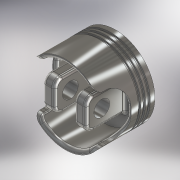
# Autodesk Inventor part: Piston head
Saved by Autodesk Inventor 2019 (Build 230136000, 136)
## iProperties
Created: 2020-05-28
Part Number: Piston head
Material: Generic
Document SubType Name: Modeling
Designer: Manoj
Density: 1 g/cm^3
Appearance: Chrome - Polished
Mass: 435.392 g
Surface Area: 893.496 cm^2
Volume: 435.392 cm^3
Author: Manoj
Autodesk Inventor part; units mm, degrees
ref_plane "YZ Plane" through (0, 0, 0) normal (1, 0, 0) x (0, 1, 0)
ref_plane "XZ Plane" through (0, 0, 0) normal (0, 1, 0) x (-1, 0, 0)
ref_plane "XY Plane" through (0, 0, 0) normal (0, 0, 1) x (1, 0, 0)
sketch "Sketch1" plane through (0, 0, 0) normal (0, 0, 1) x (1, 0, 0)
  line L0 (0, 0) -> (63.5, 0)
  line L1 (63.5, 0) -> (63.5, -81.28)
  line L2 (63.5, -81.28) -> (57.15, -81.28)
  line L3 (57.15, -81.28) -> (57.15, -19)
  line L4 (57.15, -19) -> (0, -19)
  line L5 (0, -19) -> (0, 0)
  dimension "d0" = 63.5
  dimension "d1" = 19
  dimension "d2" = 81.28
  dimension "d3" = 6.35
  constraints: 12 end point, 5 perpendicular, 1 horizontal
  measures "d0" distance of L0.start L0.end
  measures "d1" distance between parallel lines of L0 L4
  measures "d2" distance of L0.end L1.end
  measures "d3" distance of L1.end L2.end
revolve "Revolution1" add sketch "Sketch1" angle 360 about axis through (0, -19, 0) along (0, 1, 0)
sketch "Sketch2" plane through (0, 0, 0) normal (0, 0, 1) x (1, 0, 0)
  line L0 (-63.5, -81.28) -> (-63.5, 0) construction
  line L1 (-63.5, 0) -> (63.5, 0) construction
  line L2 (63.5, 0) -> (63.5, -81.28) construction
  line L3 (63.5, -81.28) -> (57.15, -81.28) construction
  line L4 (57.15, -81.28) -> (57.15, -19) construction
  line L5 (57.15, -19) -> (-57.15, -19) construction
  line L6 (-57.15, -19) -> (-57.15, -81.28) construction
  line L7 (-57.15, -81.28) -> (-63.5, -81.28) construction
  line L8 (63.5, -11.43) -> (60.96, -11.43)
  line L9 (60.96, -11.43) -> (60.96, -7.62)
  line L10 (60.96, -7.62) -> (63.5, -7.62)
  line L11 (63.5, -7.62) -> (63.5, -11.43)
  line L12 (0, -97.536) -> (0, 16.256) projected
  point P0 (0, 0)
  dimension "d5" = 3.81
  dimension "d6" = 7.62
  dimension "d7" = 2.54
  constraints: 8 end point, 2 parallel, 1 horizontal, 1 perpendicular, 1 point on line
  measures "d5" distance of L10.end L8.start
  measures "d6" distance between parallel lines of L10 L1
  measures "d7" distance of L8.start L8.end
revolve "Revolution2" cut sketch "Sketch2" angle 360 about axis through (0, -10, 0) along (0, 1, 0)
pattern_linear "Rectangular Pattern1" count 3 spacing 7.62 along (0, -1, 0) of "Revolution2"
sketch "Sketch3" plane through (0, 0, 0) normal (0, 0, 1) x (1, 0, 0)
  line L0 (-60.96, -11.43) -> (-60.96, -7.62) construction
  line L1 (-60.96, -7.62) -> (-63.5, -7.62) construction
  line L2 (-63.5, -7.62) -> (-63.5, 0) construction
  line L3 (-63.5, 0) -> (63.5, 0) construction
  line L4 (63.5, 0) -> (63.5, -7.62) construction
  line L5 (63.5, -7.62) -> (60.96, -7.62) construction
  line L6 (60.96, -7.62) -> (60.96, -11.43) construction
  line L7 (60.96, -11.43) -> (63.5, -11.43) construction
  line L8 (63.5, -11.43) -> (63.5, -15.24) construction
  line L9 (63.5, -15.24) -> (60.96, -15.24) construction
  line L10 (60.96, -15.24) -> (60.96, -19.05) construction
  line L11 (60.96, -19.05) -> (63.5, -19.05) construction
  line L12 (63.5, -19.05) -> (63.5, -22.86) construction
  line L13 (63.5, -22.86) -> (60.96, -22.86) construction
  line L14 (60.96, -22.86) -> (60.96, -26.67) construction
  line L15 (60.96, -26.67) -> (63.5, -26.67) construction
  line L16 (63.5, -26.67) -> (63.5, -81.28) construction
  line L17 (63.5, -81.28) -> (57.15, -81.28) construction
  line L18 (57.15, -81.28) -> (57.15, -19) construction
  line L19 (57.15, -19) -> (-57.15, -19) construction
  line L20 (-57.15, -19) -> (-57.15, -81.28) construction
  line L21 (-57.15, -81.28) -> (-63.5, -81.28) construction
  line L22 (-63.5, -81.28) -> (-63.5, -26.67) construction
  line L23 (-63.5, -26.67) -> (-60.96, -26.67) construction
  line L24 (-60.96, -26.67) -> (-60.96, -22.86) construction
  line L25 (-60.96, -22.86) -> (-63.5, -22.86) construction
  line L26 (-63.5, -22.86) -> (-63.5, -19.05) construction
  line L27 (-63.5, -19.05) -> (-60.96, -19.05) construction
  line L28 (-60.96, -19.05) -> (-60.96, -15.24) construction
  line L29 (-60.96, -15.24) -> (-63.5, -15.24) construction
  line L30 (-63.5, -15.24) -> (-63.5, -11.43) construction
  line L31 (-63.5, -11.43) -> (-60.96, -11.43) construction
  line L32 (-38.1, -81.28) -> (38.1, -81.28)
  line L33 (38.1, -81.28) -> (38.1, -38.1)
  line L34 (38.1, -38.1) -> (-38.1, -38.1)
  line L35 (-38.1, -38.1) -> (-38.1, -81.28)
  line L36 (-38.1, -81.28) -> (38.1, -38.1) construction
  line L37 (38.1, -81.28) -> (-38.1, -38.1) construction
  point P0 (0, 0)
  point P1 (0, -59.69)
  point P2 (0, -59.69)
  point P3 (0, 0)
  dimension "d12" = 76.2
  dimension "d13" = 38.1
  constraints: 12 end point, 4 midpoint, 2 parallel, 1 horizontal, 1 horizontal alignment, 1 perpendicular, 1 vertical alignment
  measures "d12" distance of L32.start L32.end
  measures "d13" distance between parallel lines of L3 L34
extrude "Extrusion1" cut sketch "Sketch3" along normal through all both and the other way through all
sketch "Sketch4" plane through (0, -19, 0) normal (0, -1, 0) x (1, 0, 0)
  line L0 (-25.4, 15.88) -> (25.4, 15.88)
  line L1 (25.4, 15.88) -> (25.4, 34.88)
  line L2 (25.4, 34.88) -> (-25.4, 34.88)
  line L3 (-25.4, 34.88) -> (-25.4, 15.88)
  line L4 (-25.4, 15.88) -> (25.4, 34.88) construction
  line L5 (25.4, 15.88) -> (-25.4, 34.88) construction
  point P0 (0, 0)
  point P1 (0, 25.38)
  point P2 (0, 25.38)
  dimension "d16" = 50.8
  dimension "d17" = 19
  dimension "d18" = 15.88
  constraints: 12 end point, 3 midpoint, 2 parallel, 1 horizontal, 1 perpendicular, 1 vertical alignment
  measures "d16" distance of L2.end L1.end
  measures "d17" distance of L1.end L0.end
  measures "d18" distance from line of point (0, 0) L0
extrude "Extrusion2" add sketch "Sketch4" along normal blind 63.5
mirror "Mirror1" about plane through (0, 0, 0) normal (0, 0, 1) of "Extrusion2"
fillet "Fillet1" radius 28 4 edges at (-38.1, -38.1, 46.6985) (38.1, -38.1, 46.6985) (-38.1, -38.1, -46.6985) (38.1, -38.1, -46.6985)
sketch "Sketch5" plane through (-25.4, -19, 34.88) normal (0, 0, 1) x (1, 0, 0)
  circle A0 centre (25.4, -38.1) radius 12.7
  line L0 (50.8, -63.5) -> (0, -63.5) projected
  point P0 (25.4, 19)
  point P1 (25.4, -63.5)
  dimension "d22" = 25.4
  dimension "d23" = 25.4
  constraints: 1 centre point, 1 midpoint, 1 vertical alignment
  measures "d22" diameter of A0
  measures "d23" distance from line of L0 A0.centre
extrude "Extrusion3" cut sketch "Sketch5" against normal through all
fillet "Fillet2" radius 12.7 4 edges at (-25.4, -82.5, -25.38) (25.4, -82.5, -25.38) (25.4, -82.5, 25.38) (-25.4, -82.5, 25.38)
fillet "Fillet3" radius 10 4 edges at (-38.1, -81.28, -46.6985) (38.1, -81.28, -46.6985) (38.1, -81.28, 46.6985) (-38.1, -81.28, 46.6985)
fillet "Fillet4" radius 5 45 edges at (-21.6803, -78.7803, -15.88) (0, -82.5, -15.88) (21.6803, -78.7803, -15.88) (25.4, -44.4, -15.88) (-25.4, -44.4, -15.88) (-21.6803, -78.7803, -34.88) (0, -82.5, -34.88) (21.6803, -78.7803, -34.88) (25.4, -44.4, -34.88) (-25.4, -44.4, -34.88) (-21.6803, -78.7803, 34.88) (-25.4, -44.4, 34.88) (21.6803, -78.7803, 34.88) (25.4, -44.4, 34.88) (0, -82.5, 34.88) (21.6803, -78.7803, 15.88) (25.4, -44.4, 15.88) (-21.6803, -78.7803, 15.88) (-25.4, -44.4, 15.88) (0, -82.5, 15.88) (-25.4, -19, -25.38) (-25.4, -19, 25.38) (25.4, -19, 25.38) (25.4, -19, -25.38) (0, -19, -15.88) (0, -19, 34.88) (0, -19, 15.88) (0, -19, -34.88) (-38.1, -68.69, -42.5971) (-41.8959, -79.1228, -38.8697) (-57.15, -81.28, 0) (-41.8962, -79.123, 38.8694) (-38.1, -68.69, 42.5971) (-31.1234, -47.6064, 47.9318) (0, -38.1, 57.15) (31.1236, -47.6065, 47.9317) (38.1, -68.69, 42.5971) (41.8959, -79.1228, 38.8697) (54.8408, -81.28, -16.0812) (54.8408, -81.28, 16.0812) (41.8962, -79.123, -38.8694) (38.1, -68.69, -42.5971) (31.1234, -47.6064, -47.9318) (0, -38.1, -57.15) (-31.1236, -47.6065, -47.9317)
body "Solid1"
